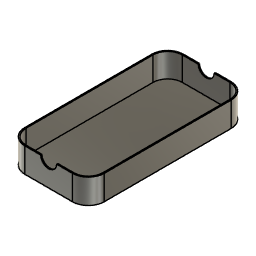
rfid botom v1 (Autodesk Fusion 360 design; units mm, degrees)
Autodesk Fusion 360 part; units mm, degrees
sketch "Sketch1" plane through (0, 0, 0) normal (0, 0, 1) x (1, 0, 0)
  line L0 (5, 0) -> (-55, 0)
  line L1 (-75, -20) -> (-75, -180)
  line L2 (-55, -200) -> (5, -200)
  line L3 (25, -180) -> (25, -20)
  arc A0 (25, -20) -> (5, 0) centre (5, -20) ccw
  arc A1 (-55, 0) -> (-75, -20) centre (-55, -20) ccw
  arc A2 (5, -200) -> (25, -180) centre (5, -180) ccw
  arc A3 (-75, -180) -> (-55, -200) centre (-55, -180) ccw
  dimension "d1" = 200
  dimension "d2" = 100
  dimension "d3" = 20
  constraint horizontal L0
  constraint vertical L1
  constraint horizontal L2
  constraint vertical L3
  constraint tangent L3 A0
  constraint tangent L0 A0
  constraint tangent L1 A1
  constraint tangent L0 A1
  constraint equal A0 A1
  constraint tangent L2 A2
  constraint tangent L3 A2
  constraint equal A0 A2
  constraint tangent L1 A3
  constraint tangent L2 A3
  constraint equal A0 A3
  measures "d1" distance of L0 L2
  measures "d2" distance of L1 L3
  measures "d3" radius of A0
extrude "Extrude1" add sketch "Sketch1" along normal blind 1
sketch "Sketch2" plane through (0, 0, 1) normal (0, 0, 1) x (-1, 0, 0)
  arc A0 (75, 180) -> (55, 200) centre (55, 180) ccw
  line L0 (55, 200) -> (-5, 200)
  arc A1 (-5, 200) -> (-25, 180) centre (-5, 180) ccw
  line L1 (-25, 180) -> (-25, 20)
  arc A2 (-25, 20) -> (-5, 0) centre (-5, 20) ccw
  line L2 (-5, 0) -> (55, 0)
  arc A3 (55, 0) -> (75, 20) centre (55, 20) ccw
  line L3 (75, 20) -> (75, 180)
  line L4 (-5, 1.5) -> (55, 1.5)
  arc A4 (55, 1.5) -> (73.5, 20) centre (55, 20) ccw
  line L5 (73.5, 20) -> (73.5, 180)
  arc A5 (73.5, 180) -> (55, 198.5) centre (55, 180) ccw
  line L6 (55, 198.5) -> (-5, 198.5)
  arc A6 (-5, 198.5) -> (-23.5, 180) centre (-5, 180) ccw
  line L7 (-23.5, 180) -> (-23.5, 20)
  arc A7 (-23.5, 20) -> (-5, 1.5) centre (-5, 20) ccw
  dimension "d6" = -1.5
extrude "Extrude2" add sketch "Sketch2" along normal blind 30
sketch "Sketch3" plane through (0, 0, 0) normal (0, 1, 0) x (-1, 0, 0)
  line L0 (-5, 0) -> (55, 0)
  line L1 (55, 0) -> (55, 31)
  line L2 (55, 31) -> (-5, 31)
  line L3 (-5, 31) -> (-5, 0)
  circle A0 centre (25, 31) radius 10
  dimension "d9" = 20
  constraint midpoint L2 A0.centre
  measures "d9" diameter of A0
extrude "Extrude3" cut sketch "Sketch3" against normal blind 10 contours L2 A0 picked at (23.7822, 27.8971)
sketch "Sketch4" plane through (0, -200, 0) normal (0, -1, 0) x (1, 0, 0)
  line L0 (-55, 0) -> (5, 0)
  line L1 (5, 0) -> (5, 31)
  line L2 (5, 31) -> (-55, 31)
  line L3 (-55, 31) -> (-55, 0)
  circle A0 centre (-25, 31) radius 10
  dimension "d12" = 20
  constraint midpoint L2 A0.centre
  measures "d12" diameter of A0
extrude "Extrude4" cut sketch "Sketch4" against normal blind 10 contours L2 A0 picked at (-26.2178, 27.8971)
